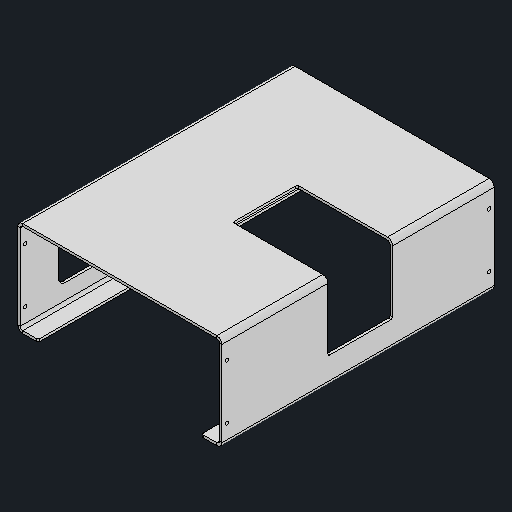
# Autodesk Inventor part: 5th Wheel Hitch Part 1
Saved by Autodesk Inventor 2025.1 (Build 291241000, 241)
## iProperties
Created: 2026-02-23
Part Number: 5th Wheel Hitch Part 1
Material: Generic
Document SubType Name: Sheet Metal
Designer: Desktop -24
Density: 1 g/cm^3
Sheet Metal Rule: Default
Appearance: Default
Author: Desktop -24
Autodesk Inventor part; units mm, degrees
ref_plane "YZ Plane" through (0, 0, 0) normal (1, 0, 0) x (0, 1, 0)
ref_plane "XZ Plane" through (0, 0, 0) normal (0, 1, 0) x (-1, 0, 0)
ref_plane "XY Plane" through (0, 0, 0) normal (0, 0, 1) x (1, 0, 0)
sketch "Sketch1" plane through (0, 0, 0) normal (0, 1, 0) x (-1, 0, 0)
  line L0 (54.705, -500) -> (-707.295, -500)
  line L1 (-707.295, 516) -> (54.705, 516)
  line L2 (54.705, 516) -> (54.705, -500)
  line L3 (-707.295, 516) -> (-707.295, -500)
  point P0 (0, 0)
  dimension "d0" = 1016
  dimension "d35" = 762
  measures "d0" distance between parallel lines of L0 L1
  measures "d35" distance of L0.start L0.end
extrude "Plate1" add sketch "Sketch1" against normal blind 9.525
sketch "Sketch6" plane through (697.77, 0, 516) normal (1, 0, 0) x (0, 1, 0)
  line L0 (0, -1016) -> (0, 0)
  line L1 (0, 0) -> (-355.6, 0)
  line L2 (-355.6, 0) -> (-355.6, -1016)
  line L3 (-355.6, -1016) -> (0, -1016)
  constraints: 6 end point, 1 horizontal, 1 perpendicular, 1 vertical
edge flange "Flange1" height 355.6 angle 90 thickness 9.525 bend radius 9.525 thickness toward (1, 0, 0) relief tear relief width 9.525 relief depth 4.7625 corner gap 9.525 corner form 0 edges at (707.295, -9.525, 8) (-54.705, -9.525, 8) wall of the first edge with corners at (697.77, 0, -500) (697.77, 0, 516) (697.77, -355.6, 516) (697.77, -355.6, -500)
bend "Bend1"
corner "Corner1"
sketch "Sketch7" plane through (707.295, -346.075, -500) normal (0, -1, 0) x (-1, 0, 0)
  line L0 (0, 1016) -> (0, 0)
  line L1 (0, 0) -> (76.2, 0)
  line L2 (76.2, 0) -> (76.2, 1016)
  line L3 (76.2, 1016) -> (0, 1016)
  constraints: 6 end point, 1 horizontal, 1 perpendicular, 1 vertical
edge flange "Flange2" height 76.2 angle 90 thickness 9.525 bend radius 9.525 thickness toward (0, -1, 0) relief tear relief width 9.525 relief depth 4.7625 corner gap 9.525 corner form 0 edges at (707.295, -355.6, 8) (-54.705, -355.6, 8) wall of the first edge with corners at (707.295, -346.075, 516) (707.295, -346.075, -500) (631.095, -346.075, -500) (631.095, -346.075, 516)
bend "Bend2"
corner "Corner2"
sketch "Sketch8" plane through (0, 0, 0) normal (0, 1, 0) x (1, 0, 0)
  line L0 (707.295, -120.65) -> (351.695, -120.65)
  line L1 (351.695, -120.65) -> (351.695, 120.65)
  line L2 (351.695, 120.65) -> (707.295, 120.65)
  line L3 (707.295, 120.65) -> (707.295, -120.65)
  line L4 (707.295, 500) -> (707.295, -516) projected
  point P0 (0, 0)
  point P1 (351.695, 0)
  dimension "d56" = 241.3
  dimension "d57" = 355.6
  constraints: 8 end point, 2 parallel, 1 horizontal, 1 horizontal alignment, 1 midpoint, 1 perpendicular, 1 point on line
  measures "d56" distance of L0.end L1.end
  measures "d57" distance of L0.start L0.end
extrude "Cut1" cut sketch "Sketch8" against normal blind 254
fillet "Corner Round4" radius 6.35 8 edges at (351.695, -4.7625, -120.65) (351.695, -4.7625, 120.65) (702.5325, -254, -120.65) (702.5325, -254, 120.65) (21.495, -350.8375, 516) (21.495, -350.8375, -500) (631.095, -350.8375, 516) (631.095, -350.8375, -500)
sketch "Sketch10" plane through (-54.705, -19.05, -500) normal (-1, 0, 0) x (0, 0, 1)
  line L0 (127, -260.35) -> (873, -260.35)
  line L1 (873, -260.35) -> (873, -57.15)
  line L2 (873, -57.15) -> (127, -57.15)
  line L3 (127, -57.15) -> (127, -260.35)
  line L4 (127, -260.35) -> (873, -57.15) construction
  line L5 (873, -260.35) -> (127, -57.15) construction
  line L6 (0, 19.05) -> (1016, 19.05) projected
  line L7 (1016, -336.55) -> (0, -336.55) projected
  line L8 (0, -317.5) -> (0, 0) projected
  point P0 (500, 19.05)
  point P1 (500, -158.75)
  dimension "d65" = 76.2
  dimension "d66" = 76.2
  dimension "d67" = 127
  constraints: 12 end point, 2 midpoint, 2 parallel, 1 horizontal, 1 perpendicular, 1 vertical alignment
  measures "d65" distance between parallel lines of L2 L6
  measures "d66" distance between parallel lines of L7 L0
  measures "d67" distance between parallel lines of L8 L3
extrude "Cut3" cut sketch "Sketch10" against normal blind 9.525
fillet "Corner Round5" radius 25.4 4 edges at (-49.9425, -279.4, -373) (-49.9425, -76.2, -373) (-49.9425, -76.2, 373) (-49.9425, -279.4, 373)
sketch "Sketch11" plane through (707.295, -336.55, 516) normal (1, 0, 0) x (0, 0, -1)
  circle A0 centre (19.05, 256.979) radius 6.35 projected
  circle A1 centre (19.05, 53.779) radius 6.35 projected
  circle A2 centre (996.95, 256.979) radius 6.35 projected
  circle A3 centre (996.95, 53.779) radius 6.35 projected
  point P0 (516, 336.55)
extrude "Cut4" cut sketch "Sketch11" against normal through all
equation "\"d68\" = Thickness"
equation "\"d71\" = Thickness"
equation "\"d10\" = Thickness"
equation "\"d36\" = BendReliefWidth"
equation "\"d37\" = BendReliefDepth"
equation "\"d38\" = MinimumRemnant"
equation "\"d39\" = TransitionRadius"
equation "\"d42\" = BendRadius"
equation "\"d43\" = CornerReliefSize"
equation "\"d44\" = GapSize"
equation "\"d45\" = JacobiRadiusSize"
equation "\"d46\" = BendReliefWidth"
equation "\"d47\" = BendReliefDepth"
equation "\"d48\" = MinimumRemnant"
equation "\"d49\" = TransitionRadius"
equation "\"d52\" = BendRadius"
equation "\"d53\" = CornerReliefSize"
equation "\"d54\" = GapSize"
equation "\"d55\" = JacobiRadiusSize"
equation "\"BendRadius\" = Thickness"
equation "\"BendReliefWidth\" = Thickness"
equation "\"BendReliefDepth\" = 0.5 * Thickness"
equation "\"CornerReliefSize\" = 4 * Thickness"
equation "\"MinimumRemnant\" = 2 * Thickness"
equation "\"TransitionRadius\" = BendRadius"
equation "\"JacobiRadiusSize\" = BendRadius"
equation "\"GapSize\" = Thickness"
equation "\"Thickness\" = 9.525"
body "Solid1"
